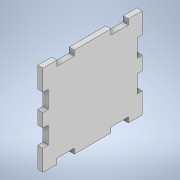
# Autodesk Inventor part: Trasera
Saved by Autodesk Inventor 2020.2 (Build 242310000, 310)
## iProperties
Created: 2020-03-18
Part Number: Trasera
Material: Generic
Document SubType Name: Modeling
Designer: ARQ SEVILLA R
Density: 1 g/cm^3
Appearance: Default
Author: ARQ SEVILLA R
Autodesk Inventor part; units mm, degrees
ref_plane "YZ Plane" through (0, 0, 0) normal (1, 0, 0) x (0, 1, 0)
ref_plane "XZ Plane" through (0, 0, 0) normal (0, 1, 0) x (-1, 0, 0)
ref_plane "XY Plane" through (0, 0, 0) normal (0, 0, 1) x (1, 0, 0)
sketch "Sketch1" plane through (0, 0, 0) normal (1, 0, 0) x (0, 1, 0)
  circle A0 centre (0, 0) radius 7.5
  line L0 (-31.75, -25.5) -> (-31.75, -20.5)
  line L1 (-31.75, -20.5) -> (-28.75, -20.5)
  line L2 (-28.75, -20.5) -> (-28.75, -10.5)
  line L3 (-28.75, -10.5) -> (-31.75, -10.5)
  line L4 (0, 0) -> (-31.75, 0) construction
  line L5 (-31.75, 20.5) -> (-28.75, 20.5)
  line L6 (-28.75, 20.5) -> (-28.75, 10.5)
  line L7 (-28.75, 10.5) -> (-31.75, 10.5)
  line L8 (-31.75, 25.5) -> (-31.75, 20.5)
  line L9 (-31.75, 10.5) -> (-31.75, -10.5)
  line L10 (-31.75, -20.5) -> (-31.75, -25.5)
  line L11 (20, 25.5) -> (20, 20.5)
  line L12 (20, 20.5) -> (17, 20.5)
  line L13 (17, 20.5) -> (17, 10.5)
  line L14 (17, 10.5) -> (20, 10.5)
  line L15 (20, -20.5) -> (17, -20.5)
  line L16 (17, -20.5) -> (17, -10.5)
  line L17 (17, -10.5) -> (20, -10.5)
  line L18 (20, 25.5) -> (20, 20.5)
  line L19 (20, 10.5) -> (20, -10.5)
  line L20 (20, -20.5) -> (20, -25.5)
  line L21 (20, 25.5) -> (20, 28.5)
  line L22 (-31.75, 28.5) -> (-31.75, 25.5)
  line L23 (-31.75, -25.5) -> (-31.75, -28.5)
  line L24 (20, -28.5) -> (20, -25.5)
  line L25 (-31.75, 28.5) -> (-19.75, 28.5)
  line L26 (-19.75, 28.5) -> (-19.75, 25.5)
  line L27 (-19.75, 25.5) -> (-9.75, 25.5)
  line L28 (-9.75, 25.5) -> (-9.75, 28.5)
  line L29 (-5.875, -28.5) -> (-5.875, 0) construction
  line L30 (8, 28.5) -> (8, 25.5)
  line L31 (8, 25.5) -> (-2, 25.5)
  line L32 (-2, 25.5) -> (-2, 28.5)
  line L33 (-19.75, -28.5) -> (-19.75, -25.5)
  line L34 (-19.75, -25.5) -> (-9.75, -25.5)
  line L35 (-9.75, -25.5) -> (-9.75, -28.5)
  line L36 (8, -25.5) -> (-2, -25.5)
  line L37 (8, -28.5) -> (8, -25.5)
  line L38 (-2, -25.5) -> (-2, -28.5)
  line L39 (-19.75, 28.5) -> (-31.75, 28.5)
  line L40 (20, 28.5) -> (8, 28.5)
  line L41 (-2, 28.5) -> (-9.75, 28.5)
  line L42 (-31.75, -28.5) -> (-19.75, -28.5)
  line L43 (-9.75, -28.5) -> (-2, -28.5)
  line L44 (8, -28.5) -> (20, -28.5)
  line L45 (-31.75, -28.5) -> (-19.75, -28.5)
  line L46 (-9.75, -28.5) -> (-5.875, -28.5)
  line L47 (-28.75, 20.5) -> (-23.5, 20.5) construction
  line L48 (-23.5, 20.5) -> (-23.5, -28.5) construction
  line L49 (-23.5, 0) -> (-23.5, -8) construction
  line L50 (-23.5, -8) -> (-20.5, -8)
  line L51 (-20.5, -8) -> (-20.5, -16)
  line L52 (-20.5, -16) -> (-23.5, -16)
  line L53 (-23.5, -8) -> (-23.5, -16)
  line L54 (-23.5, -20.5) -> (-23.5, 28.5) construction
  line L55 (-23.5, 0) -> (-23.5, 8) construction
  line L56 (-23.5, 8) -> (-20.5, 8)
  line L57 (-20.5, 8) -> (-20.5, 16)
  line L58 (-20.5, 16) -> (-23.5, 16)
  line L59 (-23.5, 8) -> (-23.5, 16)
  line L60 (0, -7.5) -> (0, -9.5) construction
  line L61 (0, -9.5) -> (1.5, -9.5)
  line L62 (1.5, -9.5) -> (1.5, -13.5)
  line L63 (1.5, -13.5) -> (-1.5, -13.5)
  line L64 (-1.5, -13.5) -> (-1.5, -9.5)
  line L65 (-1.5, -9.5) -> (0, -9.5)
  line L66 (0, 9.5) -> (1.5, 9.5)
  line L67 (1.5, 9.5) -> (1.5, 13.5)
  line L68 (1.5, 13.5) -> (-1.5, 13.5)
  line L69 (-1.5, 13.5) -> (-1.5, 9.5)
  line L70 (-1.5, 9.5) -> (0, 9.5)
  line L71 (7.5, 0) -> (9.5, 0) construction
  line L72 (9.5, 0) -> (9.5, -1.5)
  line L73 (9.5, -1.5) -> (13.5, -1.5)
  line L74 (13.5, -1.5) -> (13.5, 1.5)
  line L75 (13.5, 1.5) -> (9.5, 1.5)
  line L76 (9.5, 1.5) -> (9.5, 0)
  line L77 (-7.5, 0) -> (-9.5, 0) construction
  line L78 (-9.5, 0) -> (-9.5, -1.5)
  line L79 (-9.5, -1.5) -> (-13.5, -1.5)
  line L80 (-13.5, -1.5) -> (-13.5, 1.5)
  line L81 (-13.5, 1.5) -> (-9.5, 1.5)
  line L82 (-9.5, 1.5) -> (-9.5, 0)
  dimension "d0" = 15
  dimension "d3" = 51
  dimension "d7" = 5
  dimension "d8" = 3
  dimension "d9" = 10
  dimension "d10" = 3
  dimension "d11" = 51.75
  dimension "d12" = 3
  dimension "d13" = 3
  dimension "d14" = 12
  dimension "d15" = 3
  dimension "d16" = 10
  dimension "d17" = 25.875
  dimension "d18" = 5.25
  dimension "d19" = 8
  dimension "d20" = 3
  dimension "d21" = 8
  dimension "d22" = 2
  dimension "d23" = 1.5
  dimension "d24" = 4
  dimension "d25" = 3
  dimension "d26" = 2
  dimension "d27" = 1.5
  dimension "d28" = 4
  dimension "d29" = 3
  constraints: 166 end point, 42 perpendicular, 37 symmetric about line, 16 point on line, 3 vertical, 2 midpoint, 2 point on circle, 1 centre point, 1 coincident, 1 collinear, 1 horizontal
  measures "d0" diameter of A0
  measures "d3" distance of L11.start L20.end
  measures "d7" distance of L0.start L0.end
  measures "d8" distance of L0.end L1.end
  measures "d9" distance of L1.end L2.end
  measures "d10" distance of L11.end L12.end
  measures "d11" distance of L0.start L20.end
  measures "d12" distance of L11.start L21.end
  measures "d13" distance of L0.start L23.end
  measures "d14" distance of L22.start L25.end
  measures "d15" distance of L25.end L26.end
  measures "d16" distance of L26.end L27.end
  measures "d17" distance of L23.end L29.start
  measures "d18" distance of L6.start L47.end
  measures "d19" distance of L49.start L49.end
  measures "d20" distance of L49.end L50.end
  measures "d21" distance of L50.end L51.end
  measures "d22" distance of L60.start L60.end
  measures "d23" distance of L60.end L61.end
  measures "d24" distance of L61.end L62.end
  measures "d25" distance of L62.end L63.end
  measures "d26" distance of L71.start L71.end
  measures "d27" distance of L71.end L72.end
  measures "d28" distance of L72.end L73.end
  measures "d29" distance of L73.end L74.end
extrude "Extrusion1" add sketch "Sketch1" along normal blind 3
sketch "Sketch3" plane through (0, 0, 0) normal (-1, 0, 0) x (0, 0, 1)
  circle A0 centre (0, 0) radius 7.5
  line L0 (-13.5, -1.5) -> (-9.5, -1.5) projected
  line L1 (-9.5, -1.5) -> (-9.5, 1.5) projected
  line L2 (-9.5, -1.5) -> (-9.5, 1.5)
  line L3 (-13.5, 1.5) -> (-13.5, -1.5) projected
  line L4 (-9.5, 1.5) -> (-13.5, 1.5)
  line L5 (-13.5, 1.5) -> (-13.5, -1.5)
  line L6 (-13.5, -1.5) -> (-9.5, -1.5)
  line L7 (-1.5, 9.5) -> (1.5, 9.5) projected
  line L8 (1.5, 13.5) -> (-1.5, 13.5) projected
  line L9 (-1.5, 9.5) -> (-1.5, 13.5)
  line L10 (-1.5, 13.5) -> (1.5, 13.5)
  line L11 (1.5, 13.5) -> (1.5, 9.5)
  line L12 (1.5, 9.5) -> (-1.5, 9.5)
  line L13 (1.5, -9.5) -> (-1.5, -9.5) projected
  line L14 (-1.5, -9.5) -> (1.5, -9.5)
  line L15 (1.5, -13.5) -> (1.5, -9.5) projected
  line L16 (1.5, -9.5) -> (1.5, -13.5)
  line L17 (-1.5, -13.5) -> (1.5, -13.5) projected
  line L18 (1.5, -13.5) -> (-1.5, -13.5)
  line L19 (-1.5, -9.5) -> (-1.5, -13.5) projected
  line L20 (-1.5, -13.5) -> (-1.5, -9.5)
  line L21 (13.5, 1.5) -> (9.5, 1.5) projected
  line L22 (9.5, 1.5) -> (9.5, -1.5) projected
  line L23 (9.5, 1.5) -> (9.5, -1.5)
  line L24 (13.5, -1.5) -> (13.5, 1.5) projected
  line L25 (9.5, -1.5) -> (13.5, -1.5)
  line L26 (13.5, -1.5) -> (13.5, 1.5)
  line L27 (13.5, 1.5) -> (9.5, 1.5)
  line L28 (8, -23.5) -> (16, -23.5) projected
  line L29 (16, -20.5) -> (8, -20.5) projected
  line L30 (16, -23.5) -> (16, -20.5)
  line L31 (16, -20.5) -> (8, -20.5)
  line L32 (8, -20.5) -> (8, -23.5) projected
  line L33 (8, -20.5) -> (8, -23.5)
  line L34 (8, -23.5) -> (16, -23.5)
  line L35 (-8, -23.5) -> (-8, -20.5) projected
  line L36 (-8, -23.5) -> (-8, -20.5)
  line L37 (-8, -20.5) -> (-16, -20.5) projected
  line L38 (-8, -20.5) -> (-16, -20.5)
  line L39 (-16, -20.5) -> (-16, -23.5) projected
  line L40 (-16, -20.5) -> (-16, -23.5)
  line L41 (-16, -23.5) -> (-8, -23.5) projected
  line L42 (-16, -23.5) -> (-8, -23.5)
  constraints: 48 end point, 12 perpendicular, 8 collinear, 3 vertical, 1 centre point, 1 coincident, 1 horizontal
extrude "Extrusion2" add sketch "Sketch3" against normal up to surface (3 mm away)
body "Solid1"
